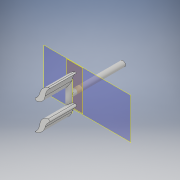
# Autodesk Inventor part: wet_proj_aandrijstang_1
Saved by Autodesk Inventor 2019.3 (Build 233278000, 278)
## iProperties
Created: 2020-03-03
Part Number: wet_proj_aandrijstang_1
Material: Generic
Document SubType Name: Modeling
Designer: Trial
Density: 1 g/cm^3
Appearance: Default
Author: Trial
Autodesk Inventor part; units mm, degrees
ref_plane "YZ Plane" through (0, 0, 0) normal (1, 0, 0) x (0, 1, 0)
ref_plane "XZ Plane" through (0, 0, 0) normal (0, 1, 0) x (-1, 0, 0)
sketch "Sketch1" plane through (0, 0, 0) normal (0, 0, 1) x (1, 0, 0)
  circle A0 centre (0, 0) radius 5
  dimension "d0" = 10
  constraints: 1 centre point, 1 coincident
  measures "d0" diameter of A0
extrude "Extrusion1" add sketch "Sketch1" along normal blind 100
sketch "Sketch2" plane through (0, 0, 0) normal (0, 1, 0) x (-1, 0, 0)
  circle A0 centre (0, 100) radius 5
  line L0 (5, 100) -> (-5, 100) projected
  point P0 (0, 0)
  dimension "d3" = 10
  constraints: 1 centre point, 1 midpoint
  measures "d3" diameter of A0
extrude "Extrusion2" add sketch "Sketch2" along normal mid plane 50
ref_plane "Work Plane1" through (0, 0, 100) normal (0, 0, 1) x (1, 0, 0)
sketch "Sketch4" plane through (0, 0, 100) normal (0, 0, 1) x (1, 0, 0)
  line L0 (5, 25) -> (-5, 25) projected
  arc A0 (14.0447, 41.8605) -> (5, 25) centre (30.3175, 22.2748) ccw
  arc A1 (10.4275, 41.7634) -> (-5, 25) centre (19.0321, 18.3637) ccw
  arc A2 (14.0447, 41.8605) -> (10.4275, 41.7634) centre (12.38, 36.4537) ccw
  arc A3 (-13.8566, 12.2457) -> (-5, 25) centre (-27.5989, 31.2405) ccw
  arc A4 (-10.2139, 9.245) -> (5, 25) centre (-12.7424, 26.9098) ccw
  arc A5 (-13.8566, 12.2457) -> (-10.2139, 9.245) centre (-10.6665, 12.407) ccw
  line L1 (110.731, 0) -> (-136.7657, 0)
  line L2 (0.0944, -80.7252) -> (0.0944, 70.6021)
  arc A6 (14.0454, -12.2457) -> (10.4026, -9.245) centre (10.8552, -12.407) ccw
  arc A7 (-10.2387, -41.7634) -> (5.1887, -25) centre (-18.8434, -18.3637) ccw
  arc A8 (-13.856, -41.8605) -> (-4.8113, -25) centre (-30.1287, -22.2748) ccw
  arc A9 (-13.856, -41.8605) -> (-10.2387, -41.7634) centre (-12.1913, -36.4537) ccw
  arc A10 (14.0454, -12.2457) -> (5.1887, -25) centre (27.7876, -31.2405) ccw
  arc A11 (10.4026, -9.245) -> (-4.8113, -25) centre (12.9311, -26.9098) ccw
  point P0 (0, 0)
  constraints: 24 point on circle, 12 centre point, 4 end point, 4 tangent, 1 horizontal, 1 vertical
ref_plane "Work Plane2" through (0, 0, 80) normal (0, 0, -1) x (-1, 0, 0)
extrude "Extrusion4" add sketch "Sketch4" along normal blind 50
ref_plane "Work Plane3" through (0, 0, 90) normal (0, 0, 1) x (1, 0, 0)
body "Solid1"
